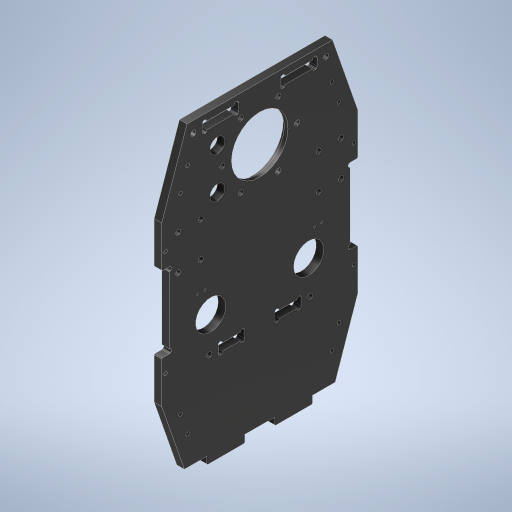
# Autodesk Inventor part: TorsoSideFrame
Saved by Autodesk Inventor 2024.2 (Build 282272000, 272)
## iProperties
Created: 2024-01-27
Part Number: TorsoSideFrame
Material: Aluminum 7075
Document SubType Name: Modeling
Designer: Masato Kubotera
Density: 2.81 g/cm^3
Appearance: Glossy - Black
Mass: 208.341 g
Surface Area: 491.779 cm^2
Volume: 74.1425 cm^3
Vendor: meviy
Author: Masato Kubotera
Autodesk Inventor part; units mm, degrees
ref_plane "YZ Plane" through (0, 0, 0) normal (1, 0, 0) x (0, 1, 0)
ref_plane "XZ Plane" through (0, 0, 0) normal (0, 1, 0) x (-1, 0, 0)
ref_plane "XY Plane" through (0, 0, 0) normal (0, 0, 1) x (1, 0, 0)
sketch "Sketch1" plane through (0, 0, 0) normal (0, 1, 0) x (-1, 0, 0)
  circle A0 centre (0, 0) radius 18.75
  line L0 (0, 0) -> (0, -161.5)
  circle A1 centre (0, 0) radius 29 construction
  line L1 (0, 0) -> (0, 36)
  line L2 (0, 36) -> (-48.2759, 36)
  line L3 (-65, -12.5) -> (-65, -106.5)
  line L4 (-50, -161.5) -> (-35, -161.5)
  line L5 (-35, -161.5) -> (-35, -166.5)
  line L6 (-35, -166.5) -> (-10, -166.5)
  line L7 (-10, -166.5) -> (-10, -161.5)
  line L8 (-10, -161.5) -> (0, -161.5)
  line L9 (-60, -40.225) -> (-65, -40.225)
  line L10 (-44, -161.5) -> (-44, -155.5) construction
  line L11 (-22.5, -166.5) -> (-22.5, -161.5) construction
  arc A2 (-7, -161.5) -> (-10, -161.5) centre (-8.5, -161.5) ccw
  arc A3 (-35, -161.5) -> (-38, -161.5) centre (-36.5, -161.5) ccw
  line L12 (-65, -12.5) -> (-60, -12.5) construction
  line L13 (-60, -12.5) -> (-60, -101.5) construction
  line L14 (-62.5, -12.5) -> (-62.5, -101.5) construction
  line L15 (-65, -40.25) -> (-60, -40.25) construction
  arc A4 (-60, -43.225) -> (-60, -40.225) centre (-60, -41.725) ccw
  line L16 (-60, -106.5) -> (0, -106.5) construction
  line L17 (-60, -101.5) -> (0, -101.5) construction
  line L18 (-60, -104) -> (-18.75, -104) construction
  line L19 (-9.95, -106.55) -> (-27.55, -106.55)
  line L20 (-27.55, -106.55) -> (-27.55, -101.45)
  line L21 (-27.55, -101.45) -> (-9.95, -101.45)
  line L22 (-9.95, -101.45) -> (-9.95, -106.55)
  line L23 (-9.95, -106.55) -> (-27.55, -101.45) construction
  line L24 (-27.55, -106.55) -> (-9.95, -101.45) construction
  line L25 (-27.5, -101.5) -> (-27.5, -106.5) construction
  arc A5 (-24.55, -101.45) -> (-27.55, -101.45) centre (-26.05, -101.45) ccw
  arc A6 (-27.55, -106.55) -> (-24.55, -106.55) centre (-26.05, -106.55) ccw
  line L26 (-22.5, -71.5) -> (-42.5, -71.5) construction
  line L27 (-42.5, -71.5) -> (-42.5, -91.5) construction
  line L28 (-42.5, -91.5) -> (-22.5, -91.5) construction
  line L29 (-22.5, -91.5) -> (-22.5, -71.5) construction
  line L30 (-22.5, -71.5) -> (-42.5, -91.5) construction
  line L31 (-42.5, -71.5) -> (-22.5, -91.5) construction
  line L32 (-45, -69) -> (-20, -69) construction
  line L33 (-20, -69) -> (-20, -94) construction
  line L34 (-20, -94) -> (-45, -94) construction
  line L35 (-45, -94) -> (-45, -69) construction
  line L36 (-45, -69) -> (-20, -94) construction
  line L37 (-20, -69) -> (-45, -94) construction
  line L38 (-50, 31) -> (0, 31) construction
  line L39 (-38.05, 31.05) -> (-13.95, 31.05)
  line L40 (-13.95, 31.05) -> (-13.95, 25.95)
  line L41 (-13.95, 25.95) -> (-38.05, 25.95)
  line L42 (-38.05, 25.95) -> (-38.05, 31.05)
  line L43 (-38.05, 31.05) -> (-13.95, 25.95) construction
  line L44 (-13.95, 31.05) -> (-38.05, 25.95) construction
  line L45 (-38.05, 28.5) -> (-13.95, 28.5) construction
  line L46 (-38, 31) -> (-38, 26) construction
  line L47 (-26, 31.05) -> (-26, 25.95) construction
  line L48 (-14, 31) -> (-14, 26) construction
  arc A7 (-35.05, 31.05) -> (-38.05, 31.05) centre (-36.55, 31.05) ccw
  arc A8 (-38.05, 25.95) -> (-35.05, 25.95) centre (-36.55, 25.95) ccw
  arc A9 (-13.95, 31.05) -> (-16.95, 31.05) centre (-15.45, 31.05) ccw
  arc A10 (-16.95, 25.95) -> (-13.95, 25.95) centre (-15.45, 25.95) ccw
  line L49 (-46.0671, -156.5) -> (-3.5, -156.5)
  arc A11 (-47.9578, -155.152) -> (-46.0671, -156.5) centre (-46.0671, -154.5) ccw
  arc A12 (-3.5, -156.5) -> (-1.5, -154.5) centre (-3.5, -154.5) ccw
  line L50 (-56, -100.25) -> (-31.1254, -100.25)
  circle A13 centre (-41.25, -65.25) radius 2 construction
  line L51 (-1.5, -63.25) -> (-56, -63.25)
  line L52 (0, 0) -> (-29, 0) construction
  line L53 (-60, -107.75) -> (-31.1254, -107.75)
  arc A14 (-29.4336, -108.6833) -> (-23.3669, -109.5167) centre (-26.05, -106.55) ccw
  line L54 (-1.5, -154.5) -> (-1.5, -109.75)
  arc A15 (-1.5, -109.75) -> (-3.5, -107.75) centre (-3.5, -109.75) ccw
  arc A16 (-29.4336, -108.6833) -> (-31.1254, -107.75) centre (-31.1254, -109.75) ccw
  circle A17 centre (-33.5, -104) radius 1.75 construction
  arc A18 (-22.0254, -109) -> (-23.3669, -109.5167) centre (-22.0254, -111) ccw
  line L55 (-18.75, -101.45) -> (-18.75, -106.55) construction
  arc A19 (-23.3669, -98.4833) -> (-29.4336, -99.3167) centre (-26.05, -101.45) ccw
  arc A20 (-31.1254, -100.25) -> (-29.4336, -99.3167) centre (-31.1254, -98.25) ccw
  arc A21 (-23.3669, -98.4833) -> (-22.0254, -99) centre (-22.0254, -97) ccw
  line L56 (-10, -101.5) -> (-10, -106.5) construction
  arc A22 (-9.95, -101.45) -> (-12.95, -101.45) centre (-11.45, -101.45) ccw
  arc A23 (-12.95, -106.55) -> (-9.95, -106.55) centre (-11.45, -106.55) ccw
  arc A24 (-14.1331, -109.5167) -> (-8.0664, -108.6833) centre (-11.45, -106.55) ccw
  arc A25 (-6.3746, -107.75) -> (-8.0664, -108.6833) centre (-6.3746, -109.75) ccw
  arc A26 (-14.1331, -109.5167) -> (-15.4746, -109) centre (-15.4746, -111) ccw
  arc A27 (-8.0664, -99.3167) -> (-6.3746, -100.25) centre (-6.3746, -98.25) ccw
  arc A28 (-8.0664, -99.3167) -> (-14.1331, -98.4833) centre (-11.45, -101.45) ccw
  arc A29 (-15.4746, -99) -> (-14.1331, -98.4833) centre (-15.4746, -97) ccw
  line L57 (-22.0254, -99) -> (-15.4746, -99)
  line L58 (-22.0254, -109) -> (-15.4746, -109)
  line L59 (-6.3746, -107.75) -> (-3.5, -107.75)
  arc A30 (-3.5, -100.25) -> (-1.5, -98.25) centre (-3.5, -98.25) ccw
  line L60 (-6.3746, -100.25) -> (-3.5, -100.25)
  line L61 (-41.25, -65.25) -> (-36.25, -65.25) construction
  line L62 (-60, -43.225) -> (-60, -87.275)
  line L63 (-60, -65.25) -> (-65, -65.25) construction
  line L64 (-60, -90.275) -> (-65, -90.275)
  line L65 (-65, -90.25) -> (-60, -90.25) construction
  arc A31 (-60, -90.275) -> (-60, -87.275) centre (-60, -88.775) ccw
  line L66 (-60, -101.5) -> (-65, -101.5) construction
  line L67 (-1.5, -22.4499) -> (-1.5, -63.25)
  line L68 (-56, -67.25) -> (-1.5, -67.25)
  line L69 (-1.5, -67.25) -> (-1.5, -98.25)
  line L70 (-56, -63.25) -> (-56, -45.4999)
  circle A32 centre (-32.5, -81.5) radius 10
  line L71 (-56, -67.25) -> (-56, -100.25)
  circle A33 centre (-32.5, -81.5) radius 11
  arc A34 (-14.0872, 17.5443) -> (-22.2374, 3.4277) centre (0, 0) ccw
  arc A35 (-22.2374, -3.4277) -> (-14.0872, -17.5443) centre (0, 0) ccw
  arc A36 (-8.1502, -20.972) -> (-1.5, -22.4499) centre (0, 0) ccw
  arc A37 (-22.2374, 3.4277) -> (-22.2374, -3.4277) centre (-24.75, 0) ccw
  line L72 (-48.2759, 36) -> (-65, -12.5)
  arc A38 (-42.9869, 36) -> (-50, 31) centre (-42.9869, 28.5817) ccw
  ellipse E0 centre (-84.0749, 16.6972) end of major axis (-93.0397, -9.3006) minor radius 20 construction
  line L73 (-75.1102, 42.6949) -> (-76.7401, 37.9681) construction
  line L74 (-105, 43.5) -> (-105, 11.4504) construction
  ellipse E1 centre (-84.0749, 16.6972) end of major axis (-76.7401, 37.9681) minor radius 15 construction
  line L75 (-75.1102, 42.6949) -> (-93.0397, -9.3006) construction
  line L76 (-84.0749, 16.6972) -> (-58.029, 7.7158) construction
  line L77 (-63.4041, 25.9649) -> (-37.3775, 16.9903) construction
  line L78 (-37.3775, 16.9903) -> (-47.4832, -12.3163) construction
  line L79 (-47.4832, -12.3163) -> (-73.5098, -3.3416) construction
  line L80 (-79.9787, 43.5) -> (-105, 43.5) construction
  line L81 (-45.1768, 19.6797) -> (-55.2826, -9.6269) construction
  circle A39 centre (-47.8663, 11.8804) radius 6.25 construction
  circle A40 centre (-52.5931, -1.8275) radius 6.25 construction
  line L82 (-1, 13.5) -> (-28, 13.5) construction
  line L83 (-28, 13.5) -> (-28, -13.5) construction
  line L84 (-28, -13.5) -> (-1, -13.5) construction
  line L85 (-1, -13.5) -> (-1, 13.5) construction
  line L86 (-1, 13.5) -> (-28, -13.5) construction
  line L87 (-28, 13.5) -> (-1, -13.5) construction
  line L88 (0, -65.25) -> (-65, -65.25) construction
  line L89 (-50, -161.5) -> (-65, -118)
  line L90 (-16.326, 23) -> (-48.5275, 23)
  arc A41 (-16.326, 23) -> (-14.0872, 17.5443) centre (-12.375, 21.4341) ccw
  line L91 (-65, -106.5) -> (-65, -118)
  arc A42 (-56, -45.4999) -> (-60, -36.225) centre (-60, -41.725) ccw
  arc A43 (-46.8371, 5.7157) -> (-50.3902, 17.5981) centre (-47.8663, 11.8804) ccw
  arc A44 (-46.8371, 5.7157) -> (-47.983, 2.3925) centre (-46.5078, 3.743) ccw
  arc A45 (-58.1048, -4.7743) -> (-47.983, 2.3925) centre (-52.5931, -1.8275) ccw
  line L92 (-48.5275, 23) -> (-50.3902, 17.5981)
  line L93 (-38, 26) -> (-14, 26) construction
  line L94 (-58.1048, -4.7743) -> (-60, -10.2703)
  line L95 (-60, -36.225) -> (-60, -10.2703)
  line L96 (-39.0921, -23.3529) -> (-39.0921, -46.6256) construction
  line L97 (-54.0921, -23.3529) -> (-54.0921, -46.6256) construction
  line L98 (-39.0921, -23.3529) -> (-54.0921, -23.3529) construction
  line L99 (-39.0921, -46.6256) -> (-54.0921, -46.6256) construction
  line L100 (-16.326, -23) -> (-48.5275, -23)
  arc A46 (-14.0872, -17.5443) -> (-16.326, -23) centre (-12.375, -21.4341) ccw
  arc A47 (-50.3902, -148.0981) -> (-46.8371, -136.2157) centre (-47.8663, -142.3804) ccw
  arc A48 (-47.983, -132.8925) -> (-46.8371, -136.2157) centre (-46.5078, -134.243) ccw
  arc A49 (-47.983, -132.8925) -> (-58.1048, -125.7257) centre (-52.5931, -128.6725) ccw
  line L101 (-47.9578, -155.152) -> (-50.3902, -148.0981)
  line L102 (-58.1048, -125.7257) -> (-60, -120.2297)
  line L103 (-60, -120.2297) -> (-60, -107.75)
  point P0 (-16.05, -9.6933)
  point P1 (-12.375, -21.4341)
  point P2 (12.375, -21.4341)
  point P3 (24.75, 0)
  point P4 (12.375, 21.4341)
  point P5 (-26, 28.5)
  point P6 (0, -130.75)
  point P7 (0, -158.0887)
  point P8 (0, -18.75)
  point P9 (0, 18.75)
  point P10 (0, -106.55)
  point P11 (-24.55, -106.55)
  point P12 (0, -101.45)
  point P13 (-35.05, 25.95)
  point P14 (-16.95, 31.05)
  point P15 (-44, 28.5)
  point P16 (-35.05, 18.95)
  point P17 (-61.4811, -94)
  point P18 (-1.5, -156.5)
  point P19 (-5, -161.5)
  point P20 (-29.8658, -107.75)
  point P21 (-30.0089, -107.1221)
  point P22 (-7.6342, -107.75)
  point P23 (-12.95, -101.45)
  point P24 (-12.95, -106.55)
  point P25 (-65, -90.275)
  point P26 (-38, 28.5)
  point P27 (-14.5, 0)
  point P28 (-1, 0)
  point P29 (-50, -161.5)
  point P30 (0, 22.5)
  point P31 (-62.5, -30.25)
  point P32 (-62.5, -100.25)
  dimension "d0" = 37.5
  dimension "d198" = 20
  dimension "d202" = 15
  dimension "d219" = 12.5
  dimension "d1" = 161.5
  dimension "d2" = 58
  dimension "d16" = 360
  dimension "d18" = 49.5
  dimension "d20" = 20
  dimension "d21" = 5
  dimension "d23" = 6
  dimension "d24" = 0.025
  dimension "d26" = 5
  dimension "d27" = 21.25
  dimension "d30" = 55
  dimension "d31" = 5
  dimension "d32" = 55
  dimension "d34" = 0.05
  dimension "d35" = 1.5
  dimension "d36" = 0.05
  dimension "d37" = 6
  dimension "d38" = 20
  dimension "d39" = 20
  dimension "d40" = 25
  dimension "d41" = 25
  dimension "d52" = 0.05
  dimension "d53" = 0.05
  dimension "d105" = 4
  dimension "d108" = 6
  dimension "d130" = 5
  dimension "d136" = 3.5
  dimension "d137" = 2
  dimension "d142" = 3
  dimension "d156" = 2.5
  dimension "d157" = 2.5
  dimension "d158" = 17.5
  dimension "d160" = 50
  dimension "d162" = 5
  dimension "d167" = 20
  dimension "d169" = 65
  dimension "d170" = 20
  dimension "d171" = 20
  dimension "d180" = 1
  dimension "d181" = 22.5
  dimension "d182" = 5
  dimension "d183" = 10
  dimension "d184" = 197.5
  dimension "d186" = 28
  dimension "d187" = 100
  dimension "d188" = 12
  dimension "d189" = 19.026
  dimension "d201" = 5
  dimension "d205" = 55
  dimension "d220" = 2
  dimension "d221" = 2
  dimension "d222" = 2
  dimension "d223" = 210
  dimension "d224" = 7.5
  dimension "d225" = 27
  dimension "d226" = 27
  dimension "d229" = 25
  dimension "d230" = 9
  dimension "d232" = 130
  dimension "d233" = 4
  dimension "d234" = 3
  dimension "d235" = 2
  dimension "d243" = 4
  dimension "d244" = 4
  constraints: 208 end point, 88 point on circle, 61 symmetric about line, 48 centre point, 43 point on line, 30 horizontal, 25 midpoint, 21 vertical, 20 tangent, 18 coincident, 15 parallel, 9 collinear, 9 equal radius, 7 perpendicular, 64 other
  measures "d1" distance of L0.start L0.end
  measures "d2" diameter of A1
  measures "d18" distance of point (24.75, 0) point (-24.75, 0)
  measures "d20" diameter of L7 L0
  measures "d21" distance of L4.end L5.end
  measures "d23" distance of L10.start L10.end
  measures "d24" distance between parallel lines of L9 L15
  measures "d26" distance of point (-36.25, -65.25) point (-41.25, -65.25)
  measures "d27" distance from line of point (-41.25, -65.25) L14
  measures "d30" distance from line of L3.end L4
  measures "d31" distance between parallel lines of L16 L17
  measures "d32" distance between parallel lines of L4 L16
  measures "d34" distance between parallel lines of L17 L21
  measures "d35" radius of A4
  measures "d36" distance between parallel lines of L20 L25
  measures "d37" distance from line of L25 point (-33.5, -104)
  measures "d38" distance of L28.end L27.end
  measures "d39" distance of L27.end L26.end
  measures "d40" distance of L33.end L34.end
  measures "d41" distance of L32.end L33.end
  measures "d52" distance between parallel lines of L42 L46
  measures "d53" distance between parallel lines of L39 L38
  measures "d105" diameter of A13
  measures "d108" distance from line of point (-44, 28.5) L46
  measures "d130" distance from line of point (-5, -161.5) L49
  measures "d136" diameter of A17
  measures "d137" distance edge to line of A17 L53
  measures "d142" diameter of L54 L0
  measures "d156" distance between parallel lines of L58 L16
  measures "d157" radial gap between concentric circles of A14 A6
  measures "d158" distance between parallel lines of L56 L25
  measures "d160" distance between parallel lines of L65 L15
  measures "d162" distance of L66.start L66.end
  measures "d167" diameter of L56 L0
  measures "d169" diameter of point (-32.5, -81.5) L0
  measures "d170" distance from line of L17 point (-32.5, -81.5)
  measures "d171" diameter of A32
  measures "d180" radial gap between concentric circles of A33 A32
  measures "d181" radius of A34
  measures "d182" distance of L46.start L46.end
  measures "d183" distance from line of L46.end L2
  measures "d184" distance between parallel lines of L2 L4
  measures "d186" diameter of L48 L1
  measures "d187" diameter of L38.start L1
  measures "d188" distance from line of L38.start L46
  measures "d189" angle of L3 L72
  measures "d201" distance of L75.start L73.end
  measures "d205" distance of L75.start L75.end
  measures "d223" diameter of L74 L1
  measures "d224" distance between parallel lines of L80 L2
  measures "d225" distance of L84.end L83.end
  measures "d226" distance of L83.end L82.end
  measures "d229" distance between parallel lines of L7 L5
  measures "d230" distance between parallel lines of L5 L10
  measures "d232" diameter of L91 L0
  measures "d233" distance between parallel lines of L72 L92
  measures "d234" distance between parallel lines of L90 L93
  measures "d235" radius of A44
  measures "d243" radial gap between concentric circles of A42 A4
extrude "Extrusion1" add sketch "Sketch1" along normal blind 5 contours A0 L0 L8 A2 L7 L6 L5 A3 L4 L89 L91 L3 L64 A31 L62 A4 L9 L72 A38 L2 L1 | A38 L72 L2 | L8 A2 | L4 A3 | A11 L101 A47 A48 A49 L102 L103 L53 A16 A14 A18 L58 A26 A24 A25 L59 A15 L54 A12 L49 | L71 L68 L69 A30 L60 A27 A28 A29 L57 A21 A19 A20 L50 | A33
extrude "Extrusion3" cut sketch "Sketch1" along normal blind 4 contours A11 L101 A47 A48 A49 L102 L103 L53 A16 A14 A18 L58 A26 A24 A25 L59 A15 L54 A12 L49 | L71 L68 L69 A30 L60 A27 A28 A29 L57 A21 A19 A20 L50
hole "M2" at (41.25, 0, -65.25) at (36.25, 0, -65.25) direction (0, 1, 0) diameter 1.567 end through all thread size "M2x0.4" class "6H" standard "ANSI Metric M Profile"
hole "M3" at (-24.75, 0, 0) at (-12.375, 0, 21.4341) at (47.8663, 0, 11.8804) at (52.5931, 0, -1.8275) at (52.5931, 0, -128.6725) at (47.8663, 0, -142.3804) at (62.5, 0, -30.25) at (62.5, 0, -100.25) direction (0, 1, 0) diameter 2.459 end through all thread size "M3x0.5" class "6H" standard "ANSI Metric M Profile"
sketch "Sketch2" plane through (65, 0, -161.5) normal (0, 0, -1) x (-1, 0, 0)
  line L0 (15, 5) -> (30, 5) projected
  line L1 (21, 5) -> (21, 0)
  line L2 (15, 0) -> (30, 0) projected
  line L3 (65, 0) -> (65, 5) projected
  point P0 (0, 5)
  point P1 (21, 0)
  point P2 (0, 0)
  point P3 (21, 2.5)
  point P4 (65, 2.5)
  constraints: 2 end point, 2 midpoint, 1 perpendicular, 1 point on line, 1 vertical
hole "Side-M3" at (44, 2.5, -161.5) at (0, 2.5, -161.5) direction (0, 0, 1) diameter 2.459 depth 6 thread size "M3x0.5" class "6H" standard "ANSI Metric M Profile"
hole "Ph3.5" at (33.5, 0, -104) at (44, 0, 28.5) at (39.0921, 0, -23.3529) at (54.0921, 0, -23.3529) at (39.0921, 0, -46.6256) at (54.0921, 0, -46.6256) direction (0, 1, 0) diameter 3.5 end through all
hole "Phi3.5-6.1" at (24.75, 0, 0) at (12.375, 0, -21.4341) at (-12.375, 0, -21.4341) at (12.375, 0, 21.4341) direction (0, 1, 0) diameter 3.5 end through all counterbore diameter 6.1 counterbore depth 3.5
hole "Phi41-H7" at (0, 0, 0) direction (0, 1, 0) diameter 41 depth 2.5
chamfer "C0.5" distance 0.5 angle 45 4 edges at (65, 2.5, -40.225) (35, 2.5, -166.5) (10, 2.5, -166.5) (65, 2.5, -90.275)
fillet "R2" radius 2.5 3 edges at (56, 2, -100.25) (1.5, 2, -67.25) (56, 2, -67.25)
mirror "Mirror1" about plane through (0, 0, 0) normal (1, 0, 0)
hole "Hole8" at (28, 0, 13.5) at (28, 0, -13.5) direction (0, 1, 0) diameter 10 end through all
body "Solid1"
